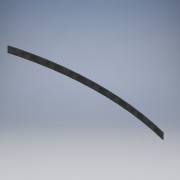
# Autodesk Inventor part: bent slat
Saved by Autodesk Inventor 2019 (Build 230136000, 136)
## iProperties
Created: 2018-08-04
Part Number: bent slat
Material: Steel
Document SubType Name: Modeling
Designer: torba
Density: 7.85 g/cm^3
Appearance: Plate
Author: torba
Autodesk Inventor part; units mm, degrees
ref_plane "YZ Plane" through (0, 0, 0) normal (1, 0, 0) x (0, 1, 0)
ref_plane "XZ Plane" through (0, 0, 0) normal (0, 1, 0) x (-1, 0, 0)
ref_plane "XY Plane" through (0, 0, 0) normal (0, 0, 1) x (1, 0, 0)
sketch "Sketch1" plane through (0, 0, 0) normal (0, 1, 0) x (-1, 0, 0)
  line L0 (73.025, 76.2127) -> (73.025, -1282.6873)
  line L1 (0, -4.7625) -> (-3.175, -4.7625)
  line L2 (-3.175, 0) -> (0, 0)
  line L3 (-3.175, -4.7625) -> (-3.175, 0)
  line L4 (3.175, 0) -> (3.175, -4.7625)
  line L5 (0, -4.7625) -> (3.175, -4.7625)
  line L6 (3.175, 0) -> (0, 0)
  line L7 (-603.2248, -75.0951) -> (-603.2248, -79.8576)
  line L8 (-609.6, -79.8576) -> (-606.3998, -79.8576)
  line L9 (-603.2248, -79.8576) -> (-606.3998, -79.8576)
  line L10 (-606.425, -75.0951) -> (-603.2248, -75.0951)
  line L11 (-606.425, -75.0951) -> (-609.6, -75.0951)
  line L12 (-609.6, -79.8576) -> (-609.6, -75.0951)
  line L13 (-1209.675, 0.0127) -> (-1209.675, -4.7498)
  line L14 (-1209.675, -4.7498) -> (-1212.85, -4.7498)
  line L15 (-1216.025, -4.7498) -> (-1212.85, -4.7498)
  line L16 (-1212.85, 0.0127) -> (-1209.675, 0.0127)
  line L17 (-1212.85, 0.0127) -> (-1216.025, 0.0127)
  line L18 (-1216.025, -4.7498) -> (-1216.025, 0.0127)
  line L19 (-1285.875, -1282.6873) -> (-1285.875, 76.2127)
  arc A0 (-1212.85, 0.0127) -> (0, 0) centre (-606.3998, 2410.819) ccw
  arc A1 (-1212.85, -4.7498) -> (0, -4.7625) centre (-606.3998, 2406.0565) ccw
  line L20 (0, 0) -> (73.025, 20.0374)
  line L21 (0, -4.7625) -> (73.025, 14.791)
  line L22 (-1212.85, 0.0127) -> (-1285.875, 20.0374)
  line L23 (-1212.85, -4.7498) -> (-1285.875, 14.791)
  dimension "d0" = 2485.9141
  dimension "d1" = 74.656
  dimension "d2" = 75.01
  dimension "d3" = 90
  dimension "d4" = 90
  dimension "d5" = 90
  dimension "d6" = 90
  dimension "d7" = 90
  dimension "d8" = 90
  dimension "d9" = 105.335
  dimension "d10" = 104.981
  dimension "d11" = 69.85
  dimension "d12" = 76.2
  dimension "d13" = 676.2498
  dimension "d14" = 682.625
  dimension "d15" = 1282.7
  dimension "d16" = 1289.05
  dimension "d17" = 1358.9
  dimension "d18" = 4.7625
  dimension "d19" = 70.3326
  dimension "d20" = 75.0951
  dimension "d21" = 0.0127
  dimension "d22" = 4.7752
  dimension "d23" = 73.025
  dimension "d24" = 0
  dimension "d25" = 4.6004
  dimension "d26" = 0
  dimension "d27" = 54.1729
  dimension "d28" = 1256.2895
  dimension "d29" = 413.7525
  dimension "d30" = 896.7099
  constraints: 48 end point, 12 parallel, 5 point on circle, 4 point on line, 3 tangent, 2 centre point, 1 equal radius, 1 horizontal, 1 vertical
  measures "d0" radius of A0
  measures "d1" angle of L20 L0
  measures "d2" angle of L0 L21
  measures "d3" angle of L6 L0
  measures "d4" angle of L5 L0
  measures "d5" angle of L9 L0
  measures "d6" angle of L0 L10
  measures "d7" angle of L17 L0
  measures "d8" angle of L15 L0
  measures "d9" angle of L0 L22
  measures "d10" angle of L0 L23
  measures "d11" distance between parallel lines of L4 L0
  measures "d12" distance between parallel lines of L3 L0
  measures "d13" distance between parallel lines of L7 L0
  measures "d14" distance between parallel lines of L12 L0
  measures "d15" distance between parallel lines of L13 L0
  measures "d16" distance between parallel lines of L18 L0
  measures "d17" distance between parallel lines of L0 L19
  measures "d18" distance between parallel lines of L2 L1
  measures "d19" distance between parallel lines of L1 L11
  measures "d20" distance between parallel lines of L1 L8
  measures "d21" distance between parallel lines of L1 L14
  measures "d22" distance between parallel lines of L1 L16
  measures "d23" distance from line of point (0, 0) L0
  measures "d24" distance from line of point (0, 0) L20
  measures "d25" distance from line of point (0, 0) L21
  measures "d26" distance from line of point (0, 0) L6
  measures "d27" distance from line of L0.start L20
  measures "d28" distance from line of L0.end L20
  measures "d29" distance from line of L19.end L20
  measures "d30" distance from line of L19.start L20
extrude "Extrusion1" add sketch "Sketch1" along normal blind 50.8 contours L0 L21 L4 L6 L20 | L6 L4 L21 L1 L3 A0 | L3 L1 A1 L7 L10 A0 | L10 L7 A1 L12 L11 | L11 L12 A1 L14 L13 A0 | L13 L14 L23 L18 L17 A0 | L15 L18 L23
body "Solid1"
